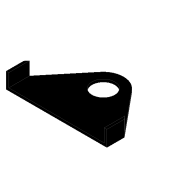
# Autodesk Inventor part: Spool Holder Stand
Saved by Autodesk Inventor 2015 (Build 190159000, 159)
## iProperties
Created: 2018-06-08
Part Number: Spool Holder Stand
Material: Generic
Document SubType Name: Modeling
Designer: Ghassan Yusuf
Density: 1 g/cm^3
Appearance: Default(2)
Author: Ghassan Yusuf
Autodesk Inventor part; units mm, degrees
ref_plane "YZ Plane" through (0, 0, 0) normal (1, 0, 0) x (0, 1, 0)
ref_plane "XZ Plane" through (0, 0, 0) normal (0, 1, 0) x (-1, 0, 0)
ref_plane "XY Plane" through (0, 0, 0) normal (0, 0, 1) x (1, 0, 0)
sketch "Sketch1" plane through (0, 0, 0) normal (0, 0, 1) x (1, 0, 0)
  circle A0 centre (0, 0) radius 26
  line L0 (-115, -107) -> (115, -107)
  arc A1 (35.4667, 29.2936) -> (-35.4667, 29.2936) centre (0, 0) ccw
  line L1 (-115, -107) -> (-115, -67)
  line L2 (-115, -107) -> (-75, -107) construction
  line L3 (115, -107) -> (115, -67)
  line L4 (115, -107) -> (155, -107) construction
  line L5 (-115, -67) -> (-35.4667, 29.2936)
  line L6 (115, -67) -> (35.4667, 29.2936)
  point P0 (0, -107)
  dimension "d0" = 52
  dimension "d2" = 107
  dimension "d3" = 230
  dimension "d4" = 20
  dimension "d5" = 40
  dimension "d6" = 90
  dimension "d7" = 40
  dimension "d8" = 90
  constraints: 14 end point, 3 horizontal, 2 centre point, 2 perpendicular, 2 point on circle, 2 tangent, 2 vertical, 1 coincident, 1 midpoint, 1 vertical alignment
  measures "d0" diameter of A0
  measures "d2" distance from line of L0 point (0, 0)
  measures "d3" distance of L0.start L0.end
  measures "d4" radial gap between concentric circles of A0 A1
  measures "d5" distance of L0.start L1.end
  measures "d6" angle of L2 L1
  measures "d7" distance of L0.end L3.end
  measures "d8" angle of L4 L3
extrude "Extrusion1" add sketch "Sketch1" along normal mid plane 6
sketch "Sketch2" plane through (0, 0, 3) normal (0, 0, 1) x (1, 0, 0)
  line L0 (-115, -107) -> (-109, -107)
  line L1 (-109, -107) -> (-109, -67)
  line L2 (-115, -67) -> (-115, -107)
  line L3 (115, -107) -> (109, -107)
  line L4 (109, -107) -> (109, -67)
  line L5 (115, -67) -> (115, -107)
  line L6 (-109, -67) -> (-109, -59.7356)
  line L7 (-35.4667, 29.2936) -> (-115, -67) projected
  line L8 (-115, -67) -> (-109, -59.7356)
  line L9 (109, -67) -> (109, -59.7356)
  line L10 (115, -67) -> (35.4667, 29.2936) projected
  line L11 (115, -67) -> (109, -59.7356)
  point P0 (0, 0)
  dimension "d12" = 6
  constraints: 20 end point, 2 collinear, 2 horizontal, 2 parallel, 2 perpendicular, 2 point on line, 2 vertical
  measures "d12" distance of L4.end L5.start
extrude "Extrusion2" add sketch "Sketch2" along normal blind 30
body "Solid1"
